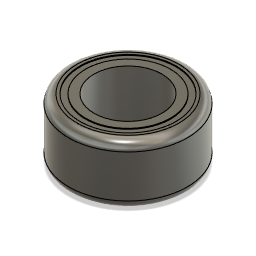
smallBearing (Autodesk Fusion 360 design; units mm, degrees)
Autodesk Fusion 360 part; units mm, degrees
note: some values were not read from the file. Set by a fixed rule: which sketch regions a step uses.
sketch "Sketch1" plane through (0, 0, 0) normal (0, 1, 0) x (1, 0, 0)
  circle A0 centre (0, 0) radius 7
  circle A1 centre (0, 0) radius 4
  dimension "d1" = 14
  dimension "d2" = 8
  constraint coincident A0.centre A1.centre
  measures "d1" diameter of A0
  measures "d2" diameter of A1
extrude "Extrude1" add sketch "Sketch1" along normal blind 7
fillet "Fillet1" radius 1 2 edges at (-6.5263, 0, 2.5313) (-6.5263, 7, 2.5313)
sketch "Sketch2" plane through (0, 7, 0) normal (0, 1, 0) x (-1, 0, 0)
  circle A0 centre (0, 0) radius 4
  circle A1 centre (0, 0) radius 6
  circle A2 centre (0, 0) radius 5.6638
  circle A3 centre (0, 0) radius 5
  constraint concentric A0 A2
  constraint concentric A0 A3
extrude "Extrude2" cut sketch "Sketch2" against normal blind 0.1 contours A2
sketch "Sketch3" plane through (0, 0, 0) normal (0, -1, 0) x (1, 0, 0)
  circle A0 centre (0, 0) radius 4
  circle A1 centre (0, 0) radius 6
  circle A2 centre (0, 0) radius 5
  circle A3 centre (0, 0) radius 5.6638
extrude "Extrude3" cut sketch "Sketch3" against normal blind 0.2 contours A3
